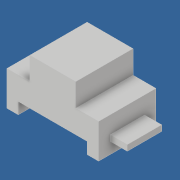
# Autodesk Inventor part: Part1
Saved by Autodesk Inventor 2018 (Build 220112000, 112)
## iProperties
Created: 2017-12-05
Part Number: Part1
Material: Generic
Document SubType Name: Modeling
Designer: 232963
Density: 1 g/cm^3
Appearance: Default
Author: 232963
Autodesk Inventor part; units mm, degrees
ref_plane "YZ Plane" through (0, 0, 0) normal (1, 0, 0) x (0, 1, 0)
ref_plane "XZ Plane" through (0, 0, 0) normal (0, 1, 0) x (-1, 0, 0)
ref_plane "XY Plane" through (0, 0, 0) normal (0, 0, 1) x (1, 0, 0)
sketch "Sketch1" plane through (0, 0, 0) normal (0, 0, 1) x (1, 0, 0)
  line L0 (40.7521, 38.1) -> (40.7521, 0)
  line L1 (-60.8479, 0) -> (-60.8479, 38.1)
  line L2 (15.3521, 38.1) -> (15.3521, 63.5)
  line L3 (15.3521, 63.5) -> (-35.4479, 63.5)
  line L4 (-35.4479, 63.5) -> (-35.4479, 38.1)
  line L5 (28.0521, 0) -> (28.0521, 12.7)
  line L6 (28.0521, 12.7) -> (-48.1479, 12.7)
  line L7 (-48.1479, 12.7) -> (-48.1479, 0)
  line L8 (40.7521, 0) -> (28.0521, 0)
  line L9 (-48.1479, 0) -> (-60.8479, 0)
  line L10 (-60.8479, 38.1) -> (-35.4479, 38.1)
  line L11 (15.3521, 38.1) -> (40.7521, 38.1)
  point P0 (0, 0)
  dimension "d4" = 101.6
  dimension "d5" = 12.7
  dimension "d6" = 12.7
  dimension "d7" = 12.7
  dimension "d8" = 38.1
  dimension "d9" = 25.4
  dimension "d10" = 25.4
  dimension "d11" = 25.4
  dimension "d12" = 25.4
  dimension "d13" = 50.8
  constraints: 24 end point, 7 parallel, 2 horizontal, 2 perpendicular
  measures "d4" distance of L0.end L1.start
  measures "d5" distance of L7.end L1.start
  measures "d6" distance of L0.end L5.start
  measures "d7" distance of L6.end L7.end
  measures "d8" distance of L1.start L1.end
  measures "d9" distance between parallel lines of L4 L1
  measures "d10" distance between parallel lines of L10 L3
  measures "d11" distance between parallel lines of L0 L2
  measures "d12" distance between parallel lines of L11 L3
  measures "d13" distance of L2.end L3.end
extrude "Extrusion1" add sketch "Sketch1" along normal blind 63.5
sketch "Sketch2" plane through (40.7521, 0, 0) normal (1, 0, 0) x (0, 0, -1)
  line L0 (-50.8, 19.05) -> (-12.7, 19.05)
  line L1 (-12.7, 19.05) -> (-12.7, 12.7)
  line L2 (-12.7, 12.7) -> (-50.8, 12.7)
  line L3 (-50.8, 12.7) -> (-50.8, 19.05)
  line L4 (0, 0) -> (0, 38.1) projected
  line L5 (0, 38.1) -> (-63.5, 38.1) projected
  dimension "d16" = 38.1
  dimension "d17" = 12.7
  dimension "d18" = 6.35
  dimension "d19" = 19.05
  constraints: 8 end point, 2 parallel, 1 horizontal, 1 perpendicular
  measures "d16" distance of L1.end L2.end
  measures "d17" distance between parallel lines of L4 L1
  measures "d18" distance of L0.end L1.end
  measures "d19" distance between parallel lines of L5 L0
extrude "Extrusion2" add sketch "Sketch2" along normal blind 19.05
body "Solid1"
